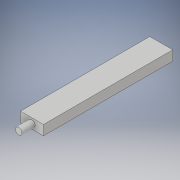
# Autodesk Inventor part: solid_for_CFD_test_06(testing device)
Saved by Autodesk Inventor 2017 (Build 210142000, 142)
## iProperties
Created: 2017-03-14
Part Number: solid_for_CFD_test_06(testing device)
Material: Generic
Document SubType Name: Modeling
Designer: XuZhiqing
Density: 1 g/cm^3
Appearance: Default
Author: XuZhiqing
Autodesk Inventor part; units mm, degrees
ref_plane "YZ Plane" through (0, 0, 0) normal (1, 0, 0) x (0, 1, 0)
ref_plane "XZ Plane" through (0, 0, 0) normal (0, 1, 0) x (-1, 0, 0)
ref_plane "XY Plane" through (0, 0, 0) normal (0, 0, 1) x (1, 0, 0)
sketch "Sketch1" plane through (0, 0, 0) normal (0, 0, 1) x (1, 0, 0)
  circle A0 centre (0, 0) radius 25.4
  dimension "d0" = 50.8
  constraints: 1 centre point, 1 coincident
  measures "d0" diameter of A0
extrude "Extrusion1" add sketch "Sketch1" along normal blind 101.6
sketch "Sketch2" plane through (0, 0, 0) normal (0, 0, 1) x (1, 0, 0)
  line L0 (88.9, 38.1) -> (-88.9, 38.1)
  line L1 (-88.9, 38.1) -> (-88.9, -38.1)
  line L2 (-88.9, -38.1) -> (88.9, -38.1)
  line L3 (88.9, -38.1) -> (88.9, 38.1)
  point P0 (0, 0)
  point P1 (0, 38.1)
  point P2 (88.9, 0)
  dimension "d3" = 76.2
  dimension "d4" = 177.8
  constraints: 8 end point, 2 midpoint, 2 parallel, 1 horizontal, 1 horizontal alignment, 1 perpendicular, 1 vertical alignment
  measures "d3" distance between parallel lines of L2 L0
  measures "d4" distance between parallel lines of L1 L3
extrude "Extrusion2" add sketch "Sketch2" against normal blind 999.998
body "Solid1"
